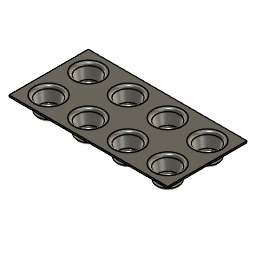
Shell Feature Specific Usecase (Autodesk Fusion 360 design; units mm, degrees)
part number: 2026-06-14-16-01-29-537
Autodesk Fusion 360 part; units mm, degrees
sketch "Sketch1" plane through (0, 0, 0) normal (0, 0, 1) x (1, 0, 0)
  line L0 (100, 50) -> (-100, 50)
  line L1 (-100, 50) -> (-100, -50)
  line L2 (-100, -50) -> (100, -50)
  line L3 (100, -50) -> (100, 50)
  line L4 (100, 50) -> (-100, -50) construction
  line L5 (-100, 50) -> (100, -50) construction
  dimension "d1" = 200
  dimension "d2" = 100
  constraint horizontal L0
  constraint perpendicular L0 L1
  constraint parallel L0 L2
  constraint parallel L1 L3
  constraint coincident L4 origin
  constraint coincident L5 origin
  measures "d1" distance of L1.end L2.end
  measures "d2" distance of L0.end L1.end
extrude "Extrude1" add sketch "Sketch1" along normal blind 30
sketch "Sketch2" plane through (0, 0, 30) normal (0, 0, 1) x (-1, 0, 0)
  line L0 (-100, 50) -> (-100, -50)
  line L1 (-100, -50) -> (100, -50)
  line L2 (100, -50) -> (100, 50)
  line L3 (100, 50) -> (-100, 50)
  circle A0 centre (75, -25) radius 15
  dimension "d5" = 30
  dimension "d6" = 25
  dimension "d7" = 25
  measures "d5" diameter of A0
  measures "d6" distance of L1 A0.centre
  measures "d7" distance of L2 A0.centre
extrude "Extrude2" cut sketch "Sketch2" against normal blind 20 draft -10 contours A0
fillet "Fillet1" radius 4 2 edges at (-61.0151, 19.5758, 30) (-64.303, 29.149, 10)
pattern_linear "R-Pattern1" count 4 spacing 50 along (1, 0, 0) count 2 spacing 50 along (0, -1, 0) of "Extrude2", "Fillet1"
shell "Shell1" thickness 2 removed faces 5 at (-33.3333, -50, 10) at (-100, 16.6667, 20) at (33.3333, 50, 10) at (100, -16.6667, 20) at (-33.3333, 16.6667, 0)
equation "d7 = d6"
